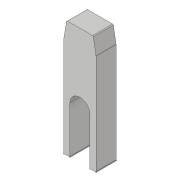
# Autodesk Inventor part: 8mm OD 6mm ID Rod Cross125
Saved by Autodesk Inventor 2017 (Build 210142000, 142)
## iProperties
Created: 2019-01-04
Part Number: 8mm OD 6mm ID Rod Cross125
Material: Generic
Document SubType Name: Sheet Metal
Designer: A. Garofalo
Density: 1 g/cm^3
Sheet Metal Rule: Default
Appearance: Default
Author: A. Garofalo
Autodesk Inventor part; units mm, degrees
ref_plane "YZ Plane" through (0, 0, 0) normal (1, 0, 0) x (0, 1, 0)
ref_plane "XZ Plane" through (0, 0, 0) normal (0, 1, 0) x (-1, 0, 0)
ref_plane "XY Plane" through (0, 0, 0) normal (0, 0, 1) x (1, 0, 0)
sketch "Sketch1" plane through (0, 0, 0) normal (0, 0, 1) x (1, 0, 0)
  line L0 (-2.54, -8.19) -> (2.54, -8.19)
  line L1 (2.54, -8.19) -> (2.54, 8.19)
  line L2 (-2.54, 8.19) -> (-2.54, -8.19)
  line L3 (-2.54, -8.19) -> (2.54, 8.19) construction
  line L4 (2.54, -8.19) -> (-2.54, 8.19) construction
  circle A0 centre (0, 16.6545) radius 2.5 construction
  circle A1 centre (0, 16.6545) radius 5
  arc A2 (6.8029, 15.0051) -> (-6.8044, 15.0114) centre (0, 16.6545) ccw
  line L5 (-2.54, 8.19) -> (-2.54, 10.2591)
  line L6 (2.54, 8.19) -> (2.54, 10.2869)
  line L7 (0, 0) -> (0, 10.7842) construction
  line L8 (-2.54, 10.2591) -> (-3.9944, 10.2511)
  line L9 (2.54, 10.2869) -> (3.9944, 10.2948)
  line L10 (-3.9944, 10.2511) -> (-4.1214, 3.9003)
  line L11 (3.9944, 10.2948) -> (4.1214, 3.9454)
  line L12 (-4.1214, 3.9003) -> (-6.8044, 15.0114)
  line L13 (4.1214, 3.9454) -> (6.8029, 15.0051)
  line L14 (0, 0) -> (0, 22.9511) construction
  point P0 (-3.2672, 10.2551)
  dimension "d2" = 5
  dimension "d3" = 10
  dimension "d4" = 14
  dimension "d8" = 1.5815
  dimension "d9" = 1.5815
  dimension "d10" = 6.35
  dimension "d11" = 6.35
  dimension "d18" = 1.4545
  dimension "d19" = 1.4545
  dimension "d31" = 2.54
  dimension "d32" = 2.54
  dimension "d33" = 0
  measures "d2" diameter of A0
  measures "d3" diameter of A1
  measures "d4" diameter of A2
  measures "d8" distance from line of L2 L10.end
  measures "d9" distance from line of L1 L11.end
  measures "d10" distance from line of L8 L10.end
  measures "d11" distance from line of L9 L11.end
  measures "d18" distance of L5.end L8.end
  measures "d19" distance of L6.end L9.end
  measures "d31" distance from line of L7.start L2
  measures "d32" distance from line of L7.start L1
  measures "d33" distance between parallel lines of L9 L8
extrude "Plate1" add sketch "Sketch1" along normal blind 3.175
sketch "Sketch2" plane through (0, 0, 0) normal (0, 0, -1) x (-1, 0, 0)
  circle A0 centre (0, 16.6545) radius 5 projected
  line L0 (-3.9944, 10.2948) -> (-4.1214, 3.9454) projected
  line L1 (-2.54, 10.2869) -> (-3.9944, 10.2948) projected
  line L2 (-2.54, -8.19) -> (-2.54, 10.2869) projected
  line L3 (2.54, -8.19) -> (-2.54, -8.19) projected
  line L4 (2.54, 10.2591) -> (2.54, -8.19) projected
  line L5 (3.9944, 10.2511) -> (2.54, 10.2591) projected
  line L6 (4.1214, 3.9003) -> (3.9944, 10.2511) projected
  line L7 (6.8044, 15.0114) -> (4.1214, 3.9003) projected
  arc A1 (6.8044, 15.0114) -> (-6.8029, 15.0051) centre (0, 16.6545) ccw projected
  line L8 (-4.1214, 3.9454) -> (-6.8029, 15.0051) projected
  line L9 (-1.5875, -17.19) -> (1.5875, -17.19)
  line L10 (1.5875, -17.19) -> (1.5875, 0.81)
  line L11 (1.5875, 0.81) -> (-1.5875, 0.81)
  line L12 (-1.5875, 0.81) -> (-1.5875, -17.19)
  line L13 (-1.5875, -17.19) -> (1.5875, 0.81) construction
  line L14 (1.5875, -17.19) -> (-1.5875, 0.81) construction
  point P0 (0, 0)
  point P1 (0, -8.19)
  dimension "d14" = 3.175
  constraints: 12 end point, 3 midpoint, 2 parallel, 1 horizontal, 1 perpendicular
  measures "d14" distance of L11.end L10.end
extrude "Extrusion1" cut sketch "Sketch2" against normal blind 25.4 contours L12 L11 L10 L3 | L3 L10 L9 L12
sketch "Sketch3" plane through (0, 0, 3.175) normal (0, 0, 1) x (1, 0, 0)
  circle A0 centre (-37.757, 0) radius 3
  line L0 (-39.3445, -2.5456) -> (-36.1695, -2.5456)
  line L1 (-36.1695, -2.5456) -> (-36.1695, 2.5456)
  line L2 (-36.1695, 2.5456) -> (-39.3445, 2.5456)
  line L3 (-39.3445, 2.5456) -> (-39.3445, -2.5456)
  line L4 (-39.3445, -2.5456) -> (-36.1695, 2.5456) construction
  line L5 (-36.1695, -2.5456) -> (-39.3445, 2.5456) construction
  circle A1 centre (-37.757, 0) radius 4
  point P0 (0, 0)
  point P1 (-37.757, 3)
  point P2 (-37.757, 4)
  dimension "d35" = 8
  dimension "d28" = 6
  dimension "d29" = 3.175
  dimension "d30" = 5.0911
  dimension "d34" = 0.4545
  dimension "d36" = 1.4545
  constraints: 12 end point, 2 midpoint, 2 parallel, 2 point on circle, 1 centre point, 1 coincident, 1 horizontal, 1 perpendicular, 1 vertical alignment, 2 other
  measures "d28" diameter of A0
  measures "d29" distance of L2.end L1.end
  measures "d30" distance of L0.end L1.end
  measures "d34" distance from line of L2 A0.end
  measures "d36" distance from line of L2 point (-37.757, 4)
sketch "Sketch4" plane through (0, 0, 3.175) normal (0, 0, 1) x (1, 0, 0)
  line L0 (-1.5875, -8.19) -> (-1.5875, 0.81) projected
  line L1 (-1.5875, 0.81) -> (1.5875, 0.81) projected
  line L2 (1.5875, 0.81) -> (1.5875, -8.19) projected
  line L3 (2.54, -8.19) -> (1.5875, -8.19) projected
  line L4 (2.54, 10.2869) -> (2.54, -8.19) projected
  line L5 (3.9944, 10.2948) -> (2.54, 10.2869) projected
  line L6 (4.1214, 3.9454) -> (3.9944, 10.2948) projected
  line L7 (6.8029, 15.0051) -> (4.1214, 3.9454) projected
  arc A0 (6.8029, 15.0051) -> (-6.8044, 15.0114) centre (0, 16.6545) ccw projected
  line L8 (-4.1214, 3.9003) -> (-6.8044, 15.0114) projected
  line L9 (-3.9944, 10.2511) -> (-4.1214, 3.9003) projected
  line L10 (-2.54, 10.2591) -> (-3.9944, 10.2511) projected
  line L11 (-2.54, -8.19) -> (-2.54, 10.2591) projected
  line L12 (-1.5875, -8.19) -> (-2.54, -8.19) projected
  circle A1 centre (0, 16.6545) radius 5 projected
  line L13 (-2.54, 10.2591) -> (-3.7175, 2.2274)
  line L14 (-3.7175, 2.2274) -> (-9.3024, 3.6769)
  line L15 (-9.3024, 3.6769) -> (-11.1796, 30.918)
  line L16 (-11.1796, 30.918) -> (24.5864, 22.2464)
  line L17 (24.5864, 22.2464) -> (4.4395, 2.4617)
  line L18 (4.4395, 2.4617) -> (3.4851, 4.2508)
  line L19 (3.4851, 4.2508) -> (2.54, 10.2869)
  line L20 (2.54, 10.2869) -> (-2.54, 10.2591)
  point P0 (0, 0)
  constraints: 16 end point
extrude "Extrusion2" cut sketch "Sketch4" against normal blind 25.4 contours L13 L14 L15 L16 L17 L18 L19 L5 L6 L7 A0 L8 L9 L10 | L10 L9 L8 A0 L7 L6 L5 L20 | A1
chamfer "Chamfer3" distance 2.54 angle 10 1 edges at (2.54, 10.2869, 1.5875) measured on face at (2.54, -2.0311, 1.0583)
chamfer "Chamfer4" distance 2.54 angle 10 1 edges at (-2.54, 10.2591, 1.5875) measured on face at (-2.54, -2.0403, 1.0583)
fillet "Fillet5" radius 0.127 4 edges at (-2.0921, 10.2615, 1.5875) (-2.54, 7.7191, 1.5875) (2.0921, 10.2844, 1.5875) (2.54, 7.7469, 1.5875)
fillet "Fillet6" radius 1.5748 2 edges at (-1.5875, 0.81, 1.5875) (1.5875, 0.81, 1.5875)
sketch "Sketch5" plane through (0, 0, 3.175) normal (0, 0, 1) x (1, 0, 0)
  arc A0 (2.54, 7.7358) -> (2.5381, 7.7578) centre (2.413, 7.7358) ccw projected
  line L0 (2.1112, 10.1789) -> (2.5381, 7.7578) projected
  arc A1 (2.1112, 10.1789) -> (1.9854, 10.2839) centre (1.9861, 10.1569) ccw projected
  line L1 (1.9854, 10.2839) -> (-1.9857, 10.2621) projected
  arc A2 (-1.9857, 10.2621) -> (-2.1101, 10.1572) centre (-1.985, 10.1351) ccw projected
  line L2 (-2.5381, 7.73) -> (-2.1101, 10.1572) projected
  arc A3 (-2.5381, 7.73) -> (-2.54, 7.708) centre (-2.413, 7.708) ccw projected
  line L3 (-2.54, -8.19) -> (-2.54, 7.708) projected
  line L4 (-1.5875, -8.19) -> (-2.54, -8.19) projected
  line L5 (-1.5875, -8.19) -> (-1.5875, -0.7648) projected
  arc A4 (-0.0127, 0.81) -> (-1.5875, -0.7648) centre (-0.0127, -0.7648) ccw projected
  line L6 (-0.0127, 0.81) -> (0.0127, 0.81) projected
  arc A5 (1.5875, -0.7648) -> (0.0127, 0.81) centre (0.0127, -0.7648) ccw projected
  line L7 (1.5875, -0.7648) -> (1.5875, -8.19) projected
  line L8 (2.54, -8.19) -> (1.5875, -8.19) projected
  line L9 (2.54, 7.7358) -> (2.54, -8.19) projected
  circle A6 centre (-2.54, -8.19) radius 0.0635
  circle A7 centre (-1.5875, -8.19) radius 0.0635
  circle A8 centre (1.5875, -8.19) radius 0.0635
  circle A9 centre (2.54, -8.19) radius 0.0635
  point P0 (0, 0)
  dimension "d48" = 0.127
  dimension "d49" = 0.127
  dimension "d50" = 0.127
  dimension "d51" = 0.127
  constraints: 4 centre point, 4 coincident
  measures "d48" diameter of A8
  measures "d49" diameter of A9
  measures "d50" diameter of A7
  measures "d51" diameter of A6
extrude "Extrusion3" add sketch "Sketch5" against normal up to surface (3.175 mm away) contours A9 L8 L9 | L9 L8 A9 | A8 L7 L8 | L8 L7 A8 | A6 L4 L3 | L3 L4 A6 | A7 L4 L5 | L5 L4 A7
fillet "Fillet7" radius 0.0508 8 edges at (-1.651, -8.19, 1.5875) (-2.4765, -8.19, 1.5875) (-2.54, -8.1265, 1.5875) (-1.5875, -8.1265, 1.5875) (2.54, -8.1265, 1.5875) (1.651, -8.19, 1.5875) (1.5875, -8.1265, 1.5875) (2.4765, -8.19, 1.5875)
equation "\"d18\" = d36"
equation "\"d19\" = d36"
equation "\"d49\" = d48"
equation "\"d50\" = d48"
equation "\"d51\" = d48"
equation "\"BendRadius\" = Thickness"
equation "\"BendReliefWidth\" = Thickness"
equation "\"BendReliefDepth\" = 0.5 * Thickness"
equation "\"CornerReliefSize\" = 4 * Thickness"
equation "\"MinimumRemnant\" = 2 * Thickness"
equation "\"TransitionRadius\" = BendRadius"
equation "\"JacobiRadiusSize\" = BendRadius"
equation "\"GapSize\" = Thickness"
equation "\"d12\" = BendRadius"
equation "\"Thickness\" = 3.175"
body "Solid1"
